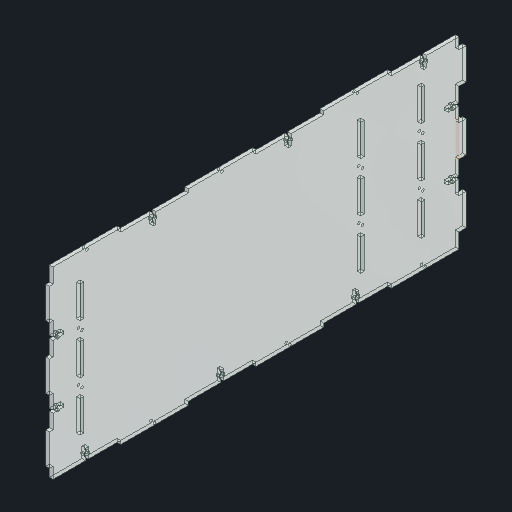
# Autodesk Inventor part: Wall
Saved by Autodesk Inventor 2024.1 (Build 281209000, 209)
## iProperties
Created: 2023-08-03
Part Number: Wall
Material: Glass
Document SubType Name: Modeling
Designer: jaege
Density: 2.18 g/cm^3
Appearance: Clear
Mass: 292.288 g
Surface Area: 1925.46 cm^2
Volume: 365.36 cm^3
Author: jaege
Autodesk Inventor part; units mm, degrees
ref_plane "YZ Plane" through (0, 0, 0) normal (1, 0, 0) x (0, 1, 0)
ref_plane "XZ Plane" through (0, 0, 0) normal (0, 1, 0) x (-1, 0, 0)
ref_plane "XY Plane" through (0, 0, 0) normal (0, 0, 1) x (1, 0, 0)
ref_plane "Work Plane1" through (87.5, -104, -4) normal (0, 1, 0) x (-1, 0, 0)
ref_plane "Work Plane2" through (-104, -17.5, -4) normal (1, 0, 0) x (0, 0, -1)
sketch "Sketch2" plane through (-104, -17.5, -4) normal (1, 0, 0) x (0, 0, -1)
  line L0 (0, 121.5) -> (0, -86.5) construction
  line L1 (0, -86.5) -> (-4, -86.5) construction
  line L2 (-4, 121.5) -> (-4, -86.5) construction
  line L3 (0, 121.5) -> (-4, 121.5) construction
  line L4 (0, -86.5) -> (0, 121.5) construction
  line L5 (0, 121.5) -> (4, 121.5) construction
  line L6 (4, -86.5) -> (4, 121.5) construction
  line L7 (0, -86.5) -> (4, -86.5) construction
  line L8 (0, -35) -> (-4, -35) projected
  line L9 (0, -35) -> (4, -35) projected
  line L10 (0, -70) -> (-4, -70) projected
  line L11 (0, -70) -> (4, -70) projected
  line L12 (0, 0) -> (4, 0) projected
  line L13 (0, 0) -> (-4, 0) projected
  line L14 (0, 35) -> (-4, 35) projected
  line L15 (0, 35) -> (4, 35) projected
  line L16 (0, 70) -> (4, 70) projected
  line L17 (0, 70) -> (-4, 70) projected
  line L18 (0, 105) -> (4, 105) projected
  line L19 (0, 105) -> (-4, 105) projected
  line L20 (4, -70) -> (4, -35)
  line L21 (4, 0) -> (4, 35)
  line L22 (4, 70) -> (4, 105)
  line L23 (-4, -70) -> (-4, -86.5)
  line L24 (-4, 105) -> (-4, 121.5)
  line L25 (-4, 70) -> (-4, 35)
  line L26 (-4, 0) -> (-4, -35)
  line L27 (-4, -86.5) -> (-454, -86.5)
  line L28 (-454, -86.5) -> (-454, 121.5)
  line L29 (-454, 121.5) -> (-4, 121.5)
  line L30 (-4, 121.5) -> (-4, -86.5)
  line L31 (-454, -70) -> (-458, -70)
  line L32 (-458, -70) -> (-458, -35)
  line L33 (-458, -35) -> (-454, -35)
  line L34 (-454, -35) -> (-454, -70)
  line L35 (-454, 0) -> (-458, 0)
  line L36 (-458, 0) -> (-458, 35)
  line L37 (-458, 35) -> (-454, 35)
  line L38 (-454, 35) -> (-454, 0)
  line L39 (-454, 70) -> (-458, 70)
  line L40 (-458, 70) -> (-458, 105)
  line L41 (-458, 105) -> (-454, 105)
  line L42 (-454, 105) -> (-454, 70)
  line L43 (-454, -86.5) -> (-379, -86.5)
  line L44 (-379, -86.5) -> (-379, -82.5)
  line L45 (-379, -82.5) -> (-454, -82.5)
  line L46 (-454, -82.5) -> (-454, -86.5)
  line L47 (-454, -86.5) -> (-379, -82.5) construction
  circle A0 centre (-416.5, -84.5) radius 1.5
  line L48 (-379, -82.5) -> (-379, -86.5)
  circle A1 centre (-341.5, -84.5) radius 1.5
  line L49 (-379, -86.5) -> (-304, -86.5)
  line L50 (-379, -86.5) -> (-304, -82.5) construction
  line L51 (-304, -86.5) -> (-304, -82.5)
  line L52 (-304, -82.5) -> (-379, -82.5)
  line L53 (-304, -82.5) -> (-304, -86.5)
  circle A2 centre (-266.5, -84.5) radius 1.5
  line L54 (-304, -86.5) -> (-229, -86.5)
  line L55 (-304, -86.5) -> (-229, -82.5) construction
  line L56 (-229, -86.5) -> (-229, -82.5)
  line L57 (-229, -82.5) -> (-304, -82.5)
  line L58 (-229, -82.5) -> (-229, -86.5)
  circle A3 centre (-191.5, -84.5) radius 1.5
  line L59 (-229, -86.5) -> (-154, -86.5)
  line L60 (-229, -86.5) -> (-154, -82.5) construction
  line L61 (-154, -86.5) -> (-154, -82.5)
  line L62 (-154, -82.5) -> (-229, -82.5)
  line L63 (-154, -82.5) -> (-154, -86.5)
  circle A4 centre (-116.5, -84.5) radius 1.5
  line L64 (-154, -86.5) -> (-79, -86.5)
  line L65 (-154, -86.5) -> (-79, -82.5) construction
  line L66 (-79, -86.5) -> (-79, -82.5)
  line L67 (-79, -82.5) -> (-154, -82.5)
  line L68 (-79, -82.5) -> (-79, -86.5)
  circle A5 centre (-41.5, -84.5) radius 1.5
  line L69 (-79, -86.5) -> (-4, -86.5)
  line L70 (-79, -86.5) -> (-4, -82.5) construction
  line L71 (-4, -86.5) -> (-4, -82.5)
  line L72 (-4, -82.5) -> (-79, -82.5)
  line L73 (-454, 121.5) -> (-454, 117.5)
  circle A6 centre (-416.5, 119.5) radius 1.5
  line L74 (-454, 117.5) -> (-379, 117.5)
  line L75 (-454, 117.5) -> (-379, 121.5) construction
  line L76 (-379, 117.5) -> (-379, 121.5)
  line L77 (-379, 121.5) -> (-454, 121.5)
  line L78 (-379, 121.5) -> (-379, 117.5)
  circle A7 centre (-341.5, 119.5) radius 1.5
  line L79 (-379, 117.5) -> (-304, 117.5)
  line L80 (-379, 117.5) -> (-304, 121.5) construction
  line L81 (-304, 117.5) -> (-304, 121.5)
  line L82 (-304, 121.5) -> (-379, 121.5)
  line L83 (-304, 121.5) -> (-304, 117.5)
  circle A8 centre (-266.5, 119.5) radius 1.5
  line L84 (-304, 117.5) -> (-229, 117.5)
  line L85 (-304, 117.5) -> (-229, 121.5) construction
  line L86 (-229, 117.5) -> (-229, 121.5)
  line L87 (-229, 121.5) -> (-304, 121.5)
  line L88 (-229, 121.5) -> (-229, 117.5)
  circle A9 centre (-191.5, 119.5) radius 1.5
  line L89 (-229, 117.5) -> (-154, 117.5)
  line L90 (-229, 117.5) -> (-154, 121.5) construction
  line L91 (-154, 117.5) -> (-154, 121.5)
  line L92 (-154, 121.5) -> (-229, 121.5)
  line L93 (-154, 121.5) -> (-154, 117.5)
  circle A10 centre (-116.5, 119.5) radius 1.5
  line L94 (-154, 117.5) -> (-79, 117.5)
  line L95 (-154, 117.5) -> (-79, 121.5) construction
  line L96 (-79, 117.5) -> (-79, 121.5)
  line L97 (-79, 121.5) -> (-154, 121.5)
  line L98 (-79, 121.5) -> (-79, 117.5)
  circle A11 centre (-41.5, 119.5) radius 1.5
  line L99 (-79, 117.5) -> (-4, 117.5)
  line L100 (-79, 117.5) -> (-4, 121.5) construction
  line L101 (-4, 117.5) -> (-4, 121.5)
  line L102 (-4, 121.5) -> (-79, 121.5)
  line L103 (-454, -19) -> (-442, -19)
  line L104 (-442, -19) -> (-442, -16)
  line L105 (-442, -16) -> (-454, -16)
  line L106 (-454, -16) -> (-454, -19)
  line L107 (-446.8, -20.2) -> (-449.2, -20.2)
  line L108 (-449.2, -20.2) -> (-449.2, -14.8)
  line L109 (-449.2, -14.8) -> (-446.8, -14.8)
  line L110 (-446.8, -14.8) -> (-446.8, -20.2)
  line L111 (-442, -17.5) -> (-454, -17.5)
  line L112 (-454, 17.5) -> (-4, 17.5) construction
  line L113 (-454, 54) -> (-442, 54)
  line L114 (-442, 54) -> (-442, 51)
  line L115 (-442, 51) -> (-454, 51)
  line L116 (-454, 51) -> (-454, 54)
  line L117 (-446.8, 55.2) -> (-449.2, 55.2)
  line L118 (-449.2, 55.2) -> (-449.2, 49.8)
  line L119 (-449.2, 49.8) -> (-446.8, 49.8)
  line L120 (-446.8, 49.8) -> (-446.8, 55.2)
  line L121 (-442, 52.5) -> (-454, 52.5)
  line L122 (-16, -19) -> (-16, -16)
  line L123 (-11.2, -14.8) -> (-11.2, -20.2)
  line L124 (-11.2, -20.2) -> (-8.8, -20.2)
  line L125 (-8.8, -20.2) -> (-8.8, -14.8)
  line L126 (-8.8, -14.8) -> (-11.2, -14.8)
  line L127 (-4, -19) -> (-16, -19)
  line L128 (-16, -17.5) -> (-4, -17.5)
  line L129 (-16, -16) -> (-4, -16)
  line L130 (-4, -16) -> (-4, -19)
  line L131 (-11.2, 55.2) -> (-8.8, 55.2)
  line L132 (-4, 54) -> (-16, 54)
  line L133 (-16, 52.5) -> (-4, 52.5)
  line L134 (-16, 54) -> (-16, 51)
  line L135 (-16, 51) -> (-4, 51)
  line L136 (-8.8, 49.8) -> (-11.2, 49.8)
  line L137 (-11.2, 49.8) -> (-11.2, 55.2)
  line L138 (-8.8, 55.2) -> (-8.8, 49.8)
  line L139 (-4, 51) -> (-4, 54)
  point P0 (-456, 70)
  point P1 (-2, 35)
  point P2 (-456, -70)
  point P3 (-454, 35)
  point P4 (-454, -82.5)
  point P5 (-379, -86.5)
  point P6 (-448, -20.2)
  point P7 (-448, -17.5)
  point P8 (-448, 55.2)
  point P9 (-448, 52.5)
  point P10 (-229, 17.5)
  point P11 (-10, -20.2)
  point P12 (-10, -17.5)
  point P13 (-10, 55.2)
  point P14 (-10, 52.5)
  point P15 (-304, -86.5)
  point P16 (-304, -82.5)
  point P17 (-229, -86.5)
  point P18 (-154, -86.5)
  point P19 (-154, -82.5)
  point P20 (-79, -86.5)
  point P21 (-4, -86.5)
  point P22 (-8.8, -19)
  point P23 (-11.2, -19)
  point P24 (-11.2, -16)
  point P25 (-8.8, -16)
  point P26 (-4, -16)
  point P27 (-4, 51)
  point P28 (-8.8, 51)
  point P29 (-11.2, 51)
  point P30 (-11.2, 54)
  point P31 (-8.8, 54)
  point P32 (-4, 121.5)
  point P33 (-79, 121.5)
  point P34 (-154, 121.5)
  point P35 (-229, 121.5)
  point P36 (-304, 121.5)
  point P37 (-379, 117.5)
  point P38 (-379, 121.5)
  point P39 (-449.2, 54)
  point P40 (-446.8, 54)
  point P41 (-446.8, 51)
  point P42 (-449.2, 51)
  point P43 (-449.2, -16)
  point P44 (-446.8, -16)
  point P45 (-446.8, -19)
  point P46 (-449.2, -19)
  point P47 (-154, -86.5)
  point P48 (-304, -86.5)
  point P49 (-304, 117.5)
  point P50 (-304, 121.5)
  point P51 (-4, 117.5)
  point P52 (-304, 117.5)
  point P53 (-379, 117.5)
  point P54 (-379, -82.5)
  point P55 (-304, -82.5)
  point P56 (-154, -82.5)
  point P57 (-4, -82.5)
  point P58 (-379, -82.5)
  point P59 (-379, -86.5)
  point P60 (-379, -86.5)
  point P61 (-4, -82.5)
  point P62 (-454, -16)
  dimension "d1" = 450
  dimension "d4" = 4
  dimension "d5" = 75
  dimension "d6" = 4
  dimension "d17" = 3
  dimension "d20" = 75
  dimension "d23" = 204
  dimension "d26" = 12
  dimension "d27" = 3
  dimension "d28" = 5.4
  dimension "d30" = 2.4
  dimension "d33" = 360
  constraints: 240 end point, 14 parallel, 12 centre point, 12 symmetric about line, 10 midpoint, 9 horizontal, 7 perpendicular, 6 horizontal alignment, 6 vertical, 5 point on line, 2 collinear, 2 vertical alignment, 209 other
  measures "d1" distance of L3.end L28.end
  measures "d4" distance between parallel lines of L32 L28
  measures "d5" distance of L45.end L44.end
  measures "d6" distance of L44.end L43.end
  measures "d17" diameter of A0
  measures "d20" distance of L27.end L48.end
  measures "d23" distance of L27.end L73.end
  measures "d26" distance of L105.end L104.end
  measures "d27" distance of L104.end L103.end
  measures "d28" distance of L109.end L107.start
  measures "d30" distance of L107.start L107.end
extrude "Extrusion1" add sketch "Sketch2" along normal blind 4 contours L9 L20 L11 L10 L30 L8 | L30 L23 L72 L67 L62 L57 L52 L45 L28 L103 L108 L107 L110 L104 L105 L109 L115 L118 L119 L120 L114 L113 L117 L74 L79 L84 L89 L94 L99 L24 L25 L132 L138 L131 L137 L134 L135 L136 L26 L129 L125 L126 L123 L122 L127 L124 | L23 L27 L66 L72 | L30 L14 L15 L21 L12 L13 | L61 L27 L56 L62 | L51 L27 L44 L52 | L30 L19 L18 L22 L16 L17 | L31 L32 L33 L28 | L94 L91 L29 L96 | L84 L81 L29 L86 | L35 L36 L37 L28 | L74 L28 L29 L76 | L28 L39 L40 L41
sketch "Sketch3" plane through (-100, -17.5, -4) normal (1, 0, 0) x (0, 0, -1)
  line L0 (-79, -86.5) -> (-4, -86.5) projected
  line L1 (-4, -86.5) -> (-4, -70) projected
  line L2 (-454, 121.5) -> (-454, 105) projected
  line L3 (-454, 105) -> (-458, 105) projected
  line L4 (-458, 105) -> (-458, 70) projected
  line L5 (-458, 70) -> (-454, 70) projected
  line L6 (-454, 70) -> (-454, 54) projected
  line L7 (-454, 0) -> (-454, -16) projected
  line L8 (-304, -86.5) -> (-304, -82.5) projected
  line L9 (-304, -82.5) -> (-229, -82.5) projected
  line L10 (-229, -82.5) -> (-229, -86.5) projected
  line L11 (-154, -86.5) -> (-154, -82.5) projected
  line L12 (-154, -82.5) -> (-79, -82.5) projected
  line L13 (-79, -82.5) -> (-79, -86.5) projected
  line L14 (-4, -70) -> (4, -70) projected
  line L15 (4, -70) -> (4, -35) projected
  line L16 (4, -35) -> (-4, -35) projected
  line L17 (-4, -35) -> (-4, -19) projected
  line L18 (-4, -19) -> (-8.8, -19) projected
  line L19 (-8.8, -19) -> (-8.8, -20.2) projected
  line L20 (-16, -16) -> (-11.2, -16) projected
  line L21 (-4, -16) -> (-4, 0) projected
  line L22 (-4, 0) -> (4, 0) projected
  line L23 (4, 0) -> (4, 35) projected
  line L24 (4, 35) -> (-4, 35) projected
  line L25 (-4, 35) -> (-4, 51) projected
  line L26 (-4, 51) -> (-8.8, 51) projected
  line L27 (-8.8, 51) -> (-8.8, 49.8) projected
  line L28 (-16, 54) -> (-11.2, 54) projected
  line L29 (-4, 54) -> (-4, 70) projected
  line L30 (-4, 70) -> (4, 70) projected
  line L31 (4, 70) -> (4, 105) projected
  line L32 (4, 105) -> (-4, 105) projected
  line L33 (-4, 105) -> (-4, 117.5) projected
  line L34 (-4, 117.5) -> (-79, 117.5) projected
  line L35 (-79, 117.5) -> (-79, 121.5) projected
  line L36 (-154, 117.5) -> (-229, 117.5) projected
  line L37 (-229, 117.5) -> (-229, 121.5) projected
  line L38 (-304, 121.5) -> (-304, 117.5) projected
  line L39 (-304, 117.5) -> (-379, 117.5) projected
  line L40 (-379, 117.5) -> (-379, 121.5) projected
  line L41 (-454, 54) -> (-449.2, 54) projected
  line L42 (-449.2, 54) -> (-449.2, 55.2) projected
  line L43 (-442, 51) -> (-446.8, 51) projected
  line L44 (-343, 117.5) -> (-340, 117.5)
  line L45 (-340, 117.5) -> (-340, 105.5)
  line L46 (-340, 105.5) -> (-343, 105.5)
  line L47 (-343, 105.5) -> (-343, 117.5)
  line L48 (-344.2, 110.3) -> (-338.8, 110.3)
  line L49 (-338.8, 110.3) -> (-338.8, 112.7)
  line L50 (-338.8, 112.7) -> (-344.2, 112.7)
  line L51 (-344.2, 112.7) -> (-344.2, 110.3)
  line L52 (-458, 17.5) -> (4, 17.5) construction
  line L53 (-190, 105.5) -> (-193, 105.5)
  line L54 (-194.2, 110.3) -> (-188.8, 110.3)
  line L55 (-188.8, 110.3) -> (-188.8, 112.7)
  line L56 (-188.8, 112.7) -> (-194.2, 112.7)
  line L57 (-194.2, 112.7) -> (-194.2, 110.3)
  line L58 (-193, 105.5) -> (-193, 117.5)
  line L59 (-190, 117.5) -> (-190, 105.5)
  line L60 (-193, 117.5) -> (-190, 117.5)
  line L61 (-40, 105.5) -> (-43, 105.5)
  line L62 (-44.2, 110.3) -> (-38.8, 110.3)
  line L63 (-38.8, 110.3) -> (-38.8, 112.7)
  line L64 (-38.8, 112.7) -> (-44.2, 112.7)
  line L65 (-44.2, 112.7) -> (-44.2, 110.3)
  line L66 (-43, 105.5) -> (-43, 117.5)
  line L67 (-40, 117.5) -> (-40, 105.5)
  line L68 (-43, 117.5) -> (-40, 117.5)
  line L69 (-418, -82.5) -> (-415, -82.5)
  line L70 (-415, -82.5) -> (-415, -70.5)
  line L71 (-415, -70.5) -> (-418, -70.5)
  line L72 (-418, -70.5) -> (-418, -82.5)
  line L73 (-419.2, -75.3) -> (-413.8, -75.3)
  line L74 (-413.8, -75.3) -> (-413.8, -77.7)
  line L75 (-413.8, -77.7) -> (-419.2, -77.7)
  line L76 (-419.2, -77.7) -> (-419.2, -75.3)
  line L77 (-454, -82.5) -> (-379, -82.5) projected
  line L78 (-229, -86.5) -> (-154, -86.5) projected
  line L79 (-79, 121.5) -> (-154, 121.5) projected
  line L80 (-154, 121.5) -> (-154, 117.5) projected
  line L81 (-229, 121.5) -> (-304, 121.5) projected
  line L82 (-379, 121.5) -> (-454, 121.5) projected
  line L83 (-454, -35) -> (-458, -35) projected
  line L84 (-458, -35) -> (-458, -70) projected
  line L85 (-458, -70) -> (-454, -70) projected
  line L86 (-454, -70) -> (-454, -82.5) projected
  line L87 (-454, -82.5) -> (-379, -82.5) projected
  line L88 (-379, -82.5) -> (-379, -86.5) projected
  line L89 (-379, -86.5) -> (-304, -86.5) projected
  line L90 (-454, 51) -> (-454, 35) projected
  line L91 (-454, 35) -> (-458, 35) projected
  line L92 (-458, 35) -> (-458, 0) projected
  line L93 (-458, 0) -> (-454, 0) projected
  line L94 (-265, -70.5) -> (-268, -70.5)
  line L95 (-269.2, -75.3) -> (-263.8, -75.3)
  line L96 (-269.2, -77.7) -> (-269.2, -75.3)
  line L97 (-263.8, -77.7) -> (-269.2, -77.7)
  line L98 (-268, -70.5) -> (-268, -82.5)
  line L99 (-268, -82.5) -> (-265, -82.5)
  line L100 (-265, -82.5) -> (-265, -70.5)
  line L101 (-263.8, -75.3) -> (-263.8, -77.7)
  line L102 (-115, -70.5) -> (-118, -70.5)
  line L103 (-119.2, -75.3) -> (-113.8, -75.3)
  line L104 (-119.2, -77.7) -> (-119.2, -75.3)
  line L105 (-113.8, -77.7) -> (-119.2, -77.7)
  line L106 (-118, -70.5) -> (-118, -82.5)
  line L107 (-118, -82.5) -> (-115, -82.5)
  line L108 (-115, -82.5) -> (-115, -70.5)
  line L109 (-113.8, -75.3) -> (-113.8, -77.7)
  line L110 (-8.8, -20.2) -> (-11.2, -20.2) projected
  line L111 (-11.2, -20.2) -> (-11.2, -19) projected
  line L112 (-11.2, -19) -> (-16, -19) projected
  line L113 (-16, -19) -> (-16, -16) projected
  line L114 (-11.2, -16) -> (-11.2, -14.8) projected
  line L115 (-11.2, -14.8) -> (-8.8, -14.8) projected
  line L116 (-8.8, -14.8) -> (-8.8, -16) projected
  line L117 (-8.8, -16) -> (-4, -16) projected
  line L118 (-8.8, 49.8) -> (-11.2, 49.8) projected
  line L119 (-11.2, 49.8) -> (-11.2, 51) projected
  line L120 (-11.2, 51) -> (-16, 51) projected
  line L121 (-16, 51) -> (-16, 54) projected
  line L122 (-11.2, 54) -> (-11.2, 55.2) projected
  line L123 (-11.2, 55.2) -> (-8.8, 55.2) projected
  line L124 (-8.8, 55.2) -> (-8.8, 54) projected
  line L125 (-8.8, 54) -> (-4, 54) projected
  line L126 (-449.2, 55.2) -> (-446.8, 55.2) projected
  line L127 (-446.8, 55.2) -> (-446.8, 54) projected
  line L128 (-446.8, 54) -> (-442, 54) projected
  line L129 (-442, 54) -> (-442, 51) projected
  line L130 (-446.8, 51) -> (-446.8, 49.8) projected
  line L131 (-446.8, 49.8) -> (-449.2, 49.8) projected
  line L132 (-449.2, 49.8) -> (-449.2, 51) projected
  line L133 (-449.2, 51) -> (-454, 51) projected
  line L134 (-454, -16) -> (-449.2, -16) projected
  line L135 (-449.2, -16) -> (-449.2, -14.8) projected
  line L136 (-449.2, -14.8) -> (-446.8, -14.8) projected
  line L137 (-446.8, -14.8) -> (-446.8, -16) projected
  line L138 (-446.8, -16) -> (-442, -16) projected
  line L139 (-442, -16) -> (-442, -19) projected
  line L140 (-442, -19) -> (-446.8, -19) projected
  line L141 (-446.8, -19) -> (-446.8, -20.2) projected
  line L142 (-446.8, -20.2) -> (-449.2, -20.2) projected
  line L143 (-449.2, -20.2) -> (-449.2, -19) projected
  line L144 (-449.2, -19) -> (-454, -19) projected
  line L145 (-454, -19) -> (-454, -35) projected
  point P0 (-4, 17.5)
  point P1 (-340, 111.5)
  point P2 (-338.8, 111.5)
  point P3 (-341.5, 112.7)
  point P4 (-341.5, 117.5)
  point P5 (-341.5, 117.5)
  point P6 (-190, 111.5)
  point P7 (-188.8, 111.5)
  point P8 (-191.5, 112.7)
  point P9 (-191.5, 117.5)
  point P10 (-191.5, 117.5)
  point P11 (-40, 111.5)
  point P12 (-38.8, 111.5)
  point P13 (-41.5, 112.7)
  point P14 (-41.5, 117.5)
  point P15 (-41.5, 117.5)
  point P16 (-413.8, -76.5)
  point P17 (-415, -76.5)
  point P18 (-416.5, -70.5)
  point P19 (-416.5, -75.3)
  point P20 (-416.5, -82.5)
  point P21 (-416.5, -82.5)
  point P22 (-416.5, -82.5)
  point P23 (-43, 110.3)
  point P24 (-40, 110.3)
  point P25 (-40, 112.7)
  point P26 (-40, 117.5)
  point P27 (-43, 117.5)
  point P28 (-43, 112.7)
  point P29 (-418, -77.7)
  point P30 (-415, -77.7)
  point P31 (-415, -75.3)
  point P32 (-418, -75.3)
  point P33 (-193, 112.7)
  point P34 (-193, 110.3)
  point P35 (-190, 110.3)
  point P36 (-190, 112.7)
  point P37 (-190, 117.5)
  point P38 (-193, 117.5)
  point P39 (-340, 112.7)
  point P40 (-340, 117.5)
  point P41 (-343, 112.7)
  point P42 (-343, 110.3)
  point P43 (-340, 110.3)
  point P44 (-416.5, -82.5)
  point P45 (-266.5, -70.5)
  point P46 (-266.5, -75.3)
  point P47 (-266.5, -82.5)
  point P48 (-265, -76.5)
  point P49 (-263.8, -76.5)
  point P50 (-266.5, -82.5)
  point P51 (-266.5, -82.5)
  point P52 (-266.5, -82.5)
  point P53 (-116.5, -70.5)
  point P54 (-116.5, -75.3)
  point P55 (-116.5, -82.5)
  point P56 (-115, -76.5)
  point P57 (-113.8, -76.5)
  point P58 (-116.5, -82.5)
  point P59 (-116.5, -82.5)
  point P60 (-116.5, -82.5)
  point P61 (-265, -75.3)
  point P62 (-268, -75.3)
  point P63 (-268, -77.7)
  point P64 (-268, -82.5)
  point P65 (-265, -82.5)
  point P66 (-265, -77.7)
  point P67 (-115, -75.3)
  point P68 (-118, -75.3)
  point P69 (-118, -77.7)
  point P70 (-118, -82.5)
  point P71 (-115, -82.5)
  point P72 (-115, -77.7)
  dimension "d35" = 2.4
  dimension "d36" = 3
  dimension "d37" = 5.4
  dimension "d38" = 12
  dimension "d41" = 150
  dimension "d60" = 150
  constraints: 98 end point, 14 midpoint, 12 parallel, 6 horizontal, 4 perpendicular, 3 coincident, 3 horizontal alignment, 2 vertical alignment, 1 point on line, 90 other
  measures "d35" distance of L50.end L48.start
  measures "d36" distance of L45.end L46.end
  measures "d37" distance of L48.start L48.end
  measures "d38" distance of L44.end L45.end
  measures "d41" distance of L46.end L53.end
  measures "d60" distance of L71.end L94.end
extrude "Extrusion2" cut sketch "Sketch3" against normal up to next contours L12 L106 L105 L108 | L108 L103 L109 L105 | L105 L106 L103 L108 | L105 L104 L103 L106 | L103 L106 L102 L108 | L9 L98 L97 L100 | L100 L95 L101 L97 | L97 L98 L95 L100 | L97 L96 L95 L98 | L95 L98 L94 L100 | L69 L72 L75 L70 | L75 L72 L73 L70 | L70 L73 L74 L75 | L75 L76 L73 L72 | L73 L72 L71 L70 | L67 L64 L66 L34 | L67 L62 L66 L64 | L64 L63 L62 L67 | L66 L62 L65 L64 | L67 L61 L66 L62 | L59 L56 L58 L36 | L59 L54 L58 L56 | L56 L55 L54 L59 | L58 L54 L57 L56 | L59 L53 L58 L54 | L45 L50 L47 L39 | L50 L49 L48 L45 | L45 L48 L47 L50 | L47 L48 L51 L50 | L45 L46 L47 L48
sketch "Sketch4" plane through (-100, -17.5, -4) normal (1, 0, 0) x (0, 0, -1)
  line L0 (-424, 90) -> (-420, 90)
  line L1 (-420, 90) -> (-420, 55)
  line L2 (-420, 55) -> (-424, 55)
  line L3 (-424, 55) -> (-424, 90)
  line L4 (-420, 0) -> (-424, 0)
  line L5 (-424, 0) -> (-424, 35)
  line L6 (-424, 35) -> (-420, 35)
  line L7 (-420, 35) -> (-420, 0)
  line L8 (-420, -20) -> (-424, -20)
  line L9 (-424, -20) -> (-424, -55)
  line L10 (-424, -55) -> (-420, -55)
  line L11 (-420, -55) -> (-420, -20)
  line L12 (-458, 35) -> (-458, 0) projected
  line L13 (-424, 55) -> (-424, 35) construction
  line L14 (-424, 0) -> (-424, -20) construction
  line L15 (-454, 121.5) -> (-454, 105) projected
  line L16 (-113, 90) -> (-109, 90)
  line L17 (-109, 90) -> (-109, 55)
  line L18 (-109, 55) -> (-113, 55)
  line L19 (-113, 55) -> (-113, 90)
  line L20 (-113, 35) -> (-109, 35)
  line L21 (-109, 35) -> (-109, 0)
  line L22 (-109, 0) -> (-113, 0)
  line L23 (-113, 0) -> (-113, 35)
  line L24 (-109, -20) -> (-113, -20)
  line L25 (-113, -20) -> (-113, -55)
  line L26 (-113, -55) -> (-109, -55)
  line L27 (-109, -55) -> (-109, -20)
  line L28 (-46, 90) -> (-42, 90)
  line L29 (-42, 90) -> (-42, 55)
  line L30 (-42, 55) -> (-46, 55)
  line L31 (-46, 55) -> (-46, 90)
  line L32 (-42, 35) -> (-46, 35)
  line L33 (-46, 35) -> (-46, 0)
  line L34 (-46, 0) -> (-42, 0)
  line L35 (-42, 0) -> (-42, 35)
  line L36 (-46, -20) -> (-42, -20)
  line L37 (-42, -20) -> (-42, -55)
  line L38 (-42, -55) -> (-46, -55)
  line L39 (-46, -55) -> (-46, -20)
  point P0 (-4, 17.5)
  point P1 (-424, 17.5)
  point P2 (-458, 17.5)
  point P3 (-422, 0)
  point P4 (-44, 90)
  point P5 (-111, 90)
  dimension "d62" = 4
  dimension "d63" = 35
  dimension "d64" = 35
  dimension "d65" = 4
  dimension "d66" = 35
  dimension "d67" = 30
  dimension "d68" = 20
  dimension "d71" = 307
  dimension "d73" = 63
  constraints: 76 end point, 18 parallel, 10 horizontal alignment, 9 horizontal, 9 perpendicular, 7 point on line, 6 equal length, 5 midpoint, 4 vertical alignment, 1 collinear
  measures "d62" distance of L1.end L2.end
  measures "d63" distance of L0.end L1.end
  measures "d64" distance of L4.end L5.end
  measures "d65" distance of L10.end L9.end
  measures "d66" distance of L9.end L8.end
  measures "d67" distance between parallel lines of L15 L3
  measures "d68" distance of L4.end L8.end
  measures "d71" distance between parallel lines of L1 L19
  measures "d73" distance of L28.start L16.end
extrude "Extrusion3" cut sketch "Sketch4" against normal up to next
sketch "Sketch5" plane through (-104, -17.5, -4) normal (-1, 0, 0) x (0, 0, 1)
  line L0 (42, 55) -> (46, 55) projected
  line L1 (42, 55) -> (46, 35) construction
  line L2 (42, 0) -> (46, 0) projected
  line L3 (46, 0) -> (42, -20) construction
  line L4 (113, 35) -> (109, 35) projected
  line L5 (109, 55) -> (113, 35) construction
  line L6 (113, 35) -> (113, 0) projected
  line L7 (109, -20) -> (109, -55) projected
  line L8 (113, 0) -> (109, -20) construction
  line L9 (420, 55) -> (424, 55) projected
  line L10 (420, 35) -> (420, 0) projected
  line L11 (424, 55) -> (420, 35) construction
  line L12 (420, 0) -> (424, -20) construction
  point P0 (4, 17.5)
  point P1 (44, 45)
  point P2 (44, -10)
  point P3 (111, 45)
  point P4 (111, -10)
  point P5 (422, -10)
  point P6 (422, 45)
  constraints: 12 end point, 6 midpoint, 1 coincident
hole "Hole1" at (-104, -27.5, 40) at (-104, 27.5, 40) at (-104, 27.5, 107) at (-104, -27.5, 107) at (-104, -27.5, 418) at (-104, 27.5, 418) direction (1, 0, 0) diameter 3 end through all
body "Solid1"
